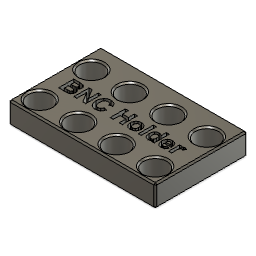
Muon BNC Holder v1 (Autodesk Fusion 360 design; units mm, degrees)
Autodesk Fusion 360 part; units mm, degrees
sketch "Sketch1" plane through (0, 0, 0) normal (0, 1, 0) x (1, 0, 0) in component "BNC Holder"
  line L0 (0, 0) -> (0, -12.75) construction
  line L1 (0, -12.75) -> (-38.25, -12.75) construction
  circle A0 centre (-38.25, -12.75) radius 7.75
  line L2 (-38.25, -12.75) -> (-38.25, 21.5) construction
  circle A1 centre (-12.75, -12.75) radius 7.75
  circle A2 centre (12.75, -12.75) radius 7.75
  circle A3 centre (38.25, -12.75) radius 7.75
  circle A4 centre (-38.25, 21.5) radius 7.75
  circle A5 centre (-12.75, 21.5) radius 7.75
  circle A6 centre (12.75, 21.5) radius 7.75
  circle A7 centre (38.25, 21.5) radius 7.75
  line L3 (0, 0) -> (0, 38) construction
  line L4 (0, 38) -> (-48.5, 38) construction
  line L5 (-48.5, 38) -> (48.5, 38)
  line L6 (48.5, 38) -> (48.5, -23)
  line L7 (48.5, -23) -> (-48.5, -23)
  line L8 (-48.5, -23) -> (-48.5, 38)
  dimension "d7" = 12.75
  dimension "d8" = 38.25
  dimension "d9" = 15.5
  dimension "d10" = 34.25
  dimension "d14" = 76.5
  dimension "d15" = 34.25
  dimension "d16" = 38
  dimension "d17" = 48.5
  dimension "d18" = 97
  dimension "d19" = 61
  constraint coincident L0.start L3.start
  constraint vertical L0
  constraint perpendicular L0 L1
  constraint coincident L1.end A0.centre
  constraint perpendicular L1 L2
  constraint parallel L0 L3
  constraint perpendicular L3 L4
  constraint horizontal L5
  constraint vertical L6
  constraint horizontal L7
  constraint vertical L8
  measures "d7" distance of L0.start L0.end
  measures "d8" distance of L0.end L1.end
  measures "d9" diameter of A0
  measures "d10" distance of L1.end L2.end
  measures "d16" distance of L0.start L3.end
  measures "d17" distance of L3.end L4.end
  measures "d18" distance of L4.end L5.end
  measures "d19" distance of L4.end L7.end
extrude "Extrude1" add sketch "Sketch1" along normal blind 14.5 in component "BNC Holder"
extrude "Extrude2" add sketch "Sketch1" along normal blind 2.5 contours A0 | A1 | A2 | A3 | A4 | A5 | A6 | A7 | L5 L6 L7 L8 in component "BNC Holder"
chamfer "Chamfer1" distance 1 angle 45 16 edges at (-45.4755, 14.5, -24.3025) (-19.9755, 14.5, -24.3025) (5.5245, 14.5, -24.3025) (31.0245, 14.5, -24.3025) (31.0245, 14.5, 9.9475) (5.5245, 14.5, 9.9475) (-19.9755, 14.5, 9.9475) (-45.4755, 14.5, 9.9475) (-48.5, 14.5, -7.5) (0, 14.5, -38) (48.5, 14.5, -7.5) (0, 14.5, 23) (48.5, 7.25, 23) (-48.5, 7.25, 23) (48.5, 7.25, -38) (-48.5, 7.25, -38) 1 faces at (-16.1667, 0, -17.6667) in component "BNC Holder"
sketch "Sketch2" plane through (0, 0, 0) normal (0, 1, 0) x (1, 0, 0) in component "BNC Holder"
  line L0 (0, 0) -> (0, 10.75) construction
  line L1 (0, 10.75) -> (-40, 10.75) construction
  line L2 (0, 0) -> (40, 0) construction
  line L3 (-40, 0) -> (40, 0) construction
  line L4 (40, 0) -> (40, 10.75) construction
  line L5 (40, 10.75) -> (-40, 10.75) construction
  line L6 (-40, 10.75) -> (-40, 0) construction
  dimension "d25" = 10.75
  dimension "d26" = 40
  dimension "d27" = 40
  dimension "d28" = 10
  text T0 "BNC Holder" font "Arial" height 10 bold align centre middle in box 80 x 10.75 at (-40, 0) x (1, 0) y (0, 1) spacing 1
  constraint coincident L0.start L2.start
  constraint vertical L0
  constraint perpendicular L0 L1
  constraint perpendicular L0 L2
  constraint coincident L2.end
  constraint coincident L1.end
  measures "d25" distance of L0.start L0.end
  measures "d26" distance of L0.end L1.end
  measures "d27" distance of L0.start L2.end
extrude "Extrude3" cut sketch "Sketch2" against normal blind 6 from surface at 14.5 text T0 in component "BNC Holder"
component "BNC Holder" placed x (1, 0, 0) y (0, 1, 0) z (0, 0, 1) at (0, 0, 0)
equation "BNCDiameter = 15.5 mm"
equation "BNCHeight = 12 mm"
equation "Spacing = 10 mm"
equation "WallThickness = 2.5 mm"
equation "SplitterLength = 33 mm"
equation "SplitterWidth = 11.5 mm"
equation "d7 = ( BNCDiameter + Spacing ) / 2"
equation "d8 = ( ( BNCDiameter + Spacing ) * 3 ) / 2"
equation "d9 = BNCDiameter"
equation "d10 = Spacing + ( BNCDiameter + SplitterLength ) / 2"
equation "d14 = BNCDiameter * 3 + Spacing * 3"
equation "d15 = ( BNCDiameter + SplitterLength ) / 2 + Spacing"
equation "d16 = SplitterLength + Spacing / 2"
equation "d17 = Spacing * 1.5 + BNCDiameter * 2 + WallThickness"
equation "d18 = Spacing * 3 + BNCDiameter * 4 + WallThickness * 2"
equation "d19 = SplitterLength + Spacing + BNCDiameter + WallThickness"
equation "d20 = WallThickness + BNCHeight"
equation "d22 = WallThickness"
equation "d25 = ( Spacing + SplitterLength ) / 4"
equation "d27 = d26"
equation "d30 = -BNCHeight / 2"
named bodies: "BNC Holder"
